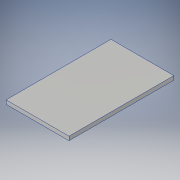
# Autodesk Inventor part: mplate
Saved by Autodesk Inventor 2019 (Build 230136000, 136)
## iProperties
Created: 2022-09-05
Part Number: mplate
Material: Aluminum 6061
Document SubType Name: Modeling
Designer: kananovicha
Density: 2.7 g/cm^3
Appearance: Aluminum - Flat
Author: kananovicha
Autodesk Inventor part; units mm, degrees
ref_plane "YZ Plane" through (0, 0, 0) normal (1, 0, 0) x (0, 1, 0)
ref_plane "XZ Plane" through (0, 0, 0) normal (0, 1, 0) x (-1, 0, 0)
ref_plane "XY Plane" through (0, 0, 0) normal (0, 0, 1) x (1, 0, 0)
sketch "Sketch1" plane through (0, 0, 0) normal (0, 0, 1) x (1, 0, 0)
  line L0 (-152.4, 9.525) -> (152.4, 9.525)
  line L1 (152.4, 9.525) -> (152.4, -9.525)
  line L2 (152.4, -9.525) -> (-152.4, -9.525)
  line L3 (-152.4, -9.525) -> (-152.4, 9.525)
  line L4 (-152.4, 9.525) -> (152.4, -9.525) construction
  line L5 (152.4, 9.525) -> (-152.4, -9.525) construction
  point P0 (0, 0)
  dimension "d0" = 304.8
  dimension "d1" = 19.05
  constraints: 12 end point, 2 midpoint, 2 parallel, 1 horizontal, 1 perpendicular
  measures "d0" distance of L1.end L2.end
  measures "d1" distance of L0.end L1.end
extrude "Extrusion1" add sketch "Sketch1" against normal blind 508
equation "\"d0\" = mp_wid"
equation "\"d1\" = mp_thick"
equation "\"d2\" = mp_len"
equation "\"mp_wid\" = 304.8"
equation "\"mp_thick\" = 19.05"
equation "\"mp_len\" = 508"
body "Solid1"
